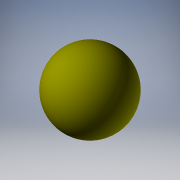
# Autodesk Inventor part: SKF_W 61710_ball1
Saved by Autodesk Inventor 2019 (Build 230136000, 136)
## iProperties
Created: 2023-04-14
Part Number: SKF_W 61710_ball1
Material: Generic
Catalog Web Link: www.cadenas.de
Description: BB1_001_101_ball1-Deep groove ball bearings
Vendor: SKF
Document SubType Name: Modeling
Designer: psAdmin
Manufacturer: SKF
Mass: 0.00706768 g
Surface Area: 0.178102 cm^2
Volume: 0.00706768 cm^3
Density: 1 g/cm^3
Appearance: PSOLRGB-175-175-175
Category: PARTsolutions
Company: SKF
Title: SKF_W 61710_ball1
Author: Cadenas PARTsolutions
Comments: Deep groove ball bearings
PSOL_IDENT_0: {$CADENAS_DATA/23d-libs/skf/bearings_units_and_housings/ball_bearings/deep_groove_ball_bearings/part
PSOL_IDENT_1: s/bb1_001_101_ball1.prj},188 {VTYP=3D},{NB=SKF_W 61710_ball1},{LINA=SKF_W 61710_ball1},{NN=BB1_001_1
PSOL_IDENT_2: 01_ball1},{DATE=25.11.2022 05:56:16},{GEOMDATE=21.11.2022 11:35:00},{VERSION=},{LINEID=17550},{WBVAR=
PSOL_IDENT_3: },{WBNUMERIC=}  {NB=SKF_W 61710_ball1},{LINA=SKF_W 61710_ball1},{KT=DUMMY},{DESIGNATION=W 61710},{R1
PSOL_IDENT_4: 2=0.30},{DD=50.000},{D=62.000},{B=6.000},{C=},{CX=},{CXX=},{CA=0.000},{XXVARIANT=},{XXDESIGN=Single
PSOL_IDENT_5: row stainless steel},{XXSEALING=No seals},{DESIGN=dgbbrs},{DESIGNIR=dgbbw},{VARIANT=},{DD1=54.30},{D
PSOL_IDENT_6: D2=},{DD2X=},{DD2A=0.00},{D1=57.80},{D1X=0.00},{D2=59.2},{D2A=59.20},{D3=},{D3X=},{D3A=0.000},{D4=},
PSOL_IDENT_7: {HH=0.000},{BB=0.000},{BBX=},{BBA=0.000},{FF=},{R0MAX=0.000},{R0=0.000},{PITCH=56.00},{DW=2.381},{DD
PSOL_IDENT_8: AMIN=52.000},{DDAMAX=0.000},{DDBMIN=0.000},{DDBMAX=0.000},{DBMIN=0.000},{DAMAX=60.000},{BBAMIN=0.000
PSOL_IDENT_9: },{CAMAX=0.000},{RAMAX=0.300},{LOAD1=1.530},{LOAD2=1.530},{LOAD3=0.067},{SPEED1=22000},{SPEED2=13000
PSOL_IDENT_10: },{KR=0.015},{F0=9.200},{Z=30},{II=1},{MASS=0.033},{BEARING=W 61710},{RING=},{HELP=2.100},{HELP2=1.4
PSOL_IDENT_11: 00},{DD1ALG=27.150},{YALG=27.150},{PITCH1=56.000},{DW1=2.381},{YALG1=28.900},{HALG1=2.100},{SH=27.15
PSOL_IDENT_12: 0},{CU=0.724},{HALG=2.15},{B1=0},{SHIELDHELP=1},{D4A=0.000},{FFA=0.000},{RS1=},{HELP3=0},{SUPPRESS=0
PSOL_IDENT_13: }
NB: SKF_W 61710_ball1
NN: BB1_001_101_ball1
NT: Deep groove ball bearings
NBSYN: SKF_$DESIGNATION._ball1
LINA: SKF_W 61710_ball1
CATALOG: SKF
DESIGNATION: W 61710
R12: 0.3
DD: 50
D: 62
B: 6
XXDESIGN: Single row stainless steel
XXSEALING: No seals
DD1: 54.3
D1: 57.8
D1X: 0
D2: 59.2
HH: 0
BB: 0
R0MAX: 0
R0: 0
PITCH: 56
DW: 2.381
DDAMIN: 52
DDAMAX: 0
DDBMIN: 0
DDBMAX: 0
DBMIN: 0
DAMAX: 60
BBAMIN: 0
CAMAX: 0
RAMAX: 0.3
LOAD1: 1.53
LOAD2: 1.53
LOAD3: 0.067
SPEED1: 22000
SPEED2: 13000
KR: 0.015
F0: 9.2
Z: 30
II: 1
MASS: 0.033
BEARING: W 61710
HELP3: 0
SUPPRESS: 0
SUPPLIER: SKF
ARTICLENO: SKF_W 61710_ball1
BOMINFO: SKF_W 61710_ball1
CREATOR: CADENAS GmbH
Autodesk Inventor part; units mm, degrees
sketch "Sketch_6" plane through (0, 0, 0) normal (0, 0, 1) x (1, 0, 0)
  line L0 (4.1905, 28) -> (1.8095, 28)
  arc A0 (4.1905, 28) -> (1.8095, 28) centre (3, 28) ccw
  line L1 (4.1905, 28) -> (1.8095, 28)
  constraints: 4 end point, 2 point on circle, 1 centre point
revolve "Revolution1" add sketch "Sketch_6" angle 360 about axis through (4.1905, 28, 0) along (1, 0, 0)
ref_plane "ball1_XY" through (3, 28, 0) normal (1, 0, 0) x (0, 0, -1)
ref_plane "ball1_YZ" through (3, 28, 0) normal (0, 0, -1) x (0, 1, 0)
ref_plane "ball1_ZX" through (3, 28, 0) normal (0, 1, 0) x (1, 0, 0)
body "Solid1"
